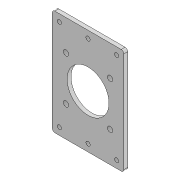
# Autodesk Inventor part: CCM_Motor_Mount_B
Saved by Autodesk Inventor 2020 (Build 240168000, 168)
## iProperties
Created: 2021-12-08
Part Number: CCM_Motor_Mount_B
Material: 一般
Document SubType Name: Sheet Metal
Designer: magnarecta
Density: 1 g/cm^3
Sheet Metal Rule: Default_mm
Appearance: 既定
Author: magnarecta
Autodesk Inventor part; units mm, degrees
ref_plane "YZ Plane" through (0, 0, 0) normal (1, 0, 0) x (0, 1, 0)
ref_plane "XZ Plane" through (0, 0, 0) normal (0, 1, 0) x (-1, 0, 0)
ref_plane "XY Plane" through (0, 0, 0) normal (0, 0, 1) x (1, 0, 0)
sketch "スケッチ1" plane through (0, 0, 0) normal (0, 0, 1) x (1, 0, 0)
  line L0 (27.5, -40.5) -> (-27.5, -40.5)
  line L1 (-27.5, -40.5) -> (-27.5, 40.5)
  line L2 (-27.5, 40.5) -> (27.5, 40.5)
  line L3 (27.5, 40.5) -> (27.5, -40.5)
  line L4 (27.5, -40.5) -> (-27.5, 40.5) construction
  line L5 (-27.5, -40.5) -> (27.5, 40.5) construction
  point P0 (0, 0)
  dimension "d0" = 55
  dimension "d1" = 81
  measures "d0" distance of L1.end L2.end
  measures "d1" distance of L0.end L1.end
extrude "プレート1" add sketch "スケッチ1" along normal blind 3
sketch "スケッチ2" plane through (0, 0, 3) normal (0, 0, 1) x (1, 0, 0)
  line L0 (-27.5, -40.5) -> (-27.5, 40.5) projected
  line L1 (27.5, -40.5) -> (-27.5, -40.5) projected
  line L2 (27.5, 40.5) -> (27.5, -40.5) projected
  line L3 (-27.5, 40.5) -> (27.5, 40.5) projected
  line L4 (22, 35) -> (22, -35)
  line L5 (22, -35) -> (-22, -35)
  line L6 (-22, -35) -> (-22, 35)
  line L7 (-22, 35) -> (22, 35)
  point P0 (0, 0)
  point P1 (0, 35)
  point P2 (0, -35)
  dimension "d3" = 5.5
  constraints: 8 end point, 4 coincident, 2 midpoint, 3 other
  measures "d3" distance between parallel lines of L3 L7
hole "穴1" at (0, 35, 3) at (0, -35, 3) at (-22, -35, 3) at (22, -35, 3) at (-22, 35, 3) at (22, 35, 3) direction (0, 0, -1) diameter 3.242 end through all thread size "M4x0.7" class "6H" standard "ISO Metric profile"
sketch "スケッチ3" plane through (0, 0, 3) normal (0, 0, 1) x (1, 0, 0)
  circle A0 centre (0, 0) radius 16.1
  dimension "d11" = 32.2
  constraints: 1 centre point, 1 coincident
  measures "d11" diameter of A0
extrude "押し出し1" cut sketch "スケッチ3" against normal blind 10
sketch "スケッチ4" plane through (0, 0, 3) normal (0, 0, 1) x (1, 0, 0)
  circle A0 centre (0, 0) radius 24
  point P0 (-16.9706, 16.9706)
  point P1 (-16.9706, -16.9706)
  point P2 (16.9706, -16.9706)
  point P3 (16.9706, 16.9706)
  dimension "d14" = 48
  dimension "d17" = 360
  constraints: 1 coincident, 1 horizontal alignment, 8 other
hole "穴2" at (-16.9706, 16.9706, 3) at (-16.9706, -16.9706, 3) at (16.9706, -16.9706, 3) at (16.9706, 16.9706, 3) direction (0, 0, -1) diameter 4.134 end through all thread size "M5x0.8" class "6H" standard "ISO Metric profile"
fillet "フィレット1" radius 2 4 edges at (-27.5, -40.5, 1.5) (27.5, -40.5, 1.5) (-27.5, 40.5, 1.5) (27.5, 40.5, 1.5)
equation "\"d2\" = Thickness"
equation "\"BendRadius\" = Thickness"
equation "\"BendReliefWidth\" = Thickness"
equation "\"BendReliefDepth\" = 0.5 * Thickness"
equation "\"CornerReliefSize\" = 4 * Thickness"
equation "\"MinimumRemnant\" = 2 * Thickness"
equation "\"TransitionRadius\" = BendRadius"
equation "\"JacobiRadiusSize\" = BendRadius"
equation "\"GapSize\" = Thickness"
equation "\"Thickness\" = 3"
